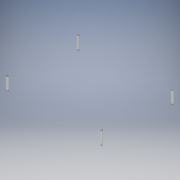
# Autodesk Inventor part: ALU
Saved by Autodesk Inventor 2019 (Build 230136000, 136)
## iProperties
Created: 2020-11-06
Part Number: ALU
Material: Generic
Document SubType Name: Modeling
Designer: james
Density: 1 g/cm^3
Appearance: Default
Author: james
Autodesk Inventor part; units mm, degrees
ref_plane "YZ Plane" through (0, 0, 0) normal (1, 0, 0) x (0, 1, 0)
ref_plane "XZ Plane" through (0, 0, 0) normal (0, 1, 0) x (-1, 0, 0)
ref_plane "XY Plane" through (0, 0, 0) normal (0, 0, 1) x (1, 0, 0)
sketch "Sketch1" plane through (0, 0, 0) normal (0, 1, 0) x (-1, 0, 0)
  line L0 (0, 0) -> (200, 0)
  line L1 (200, 0) -> (200, 152)
  line L2 (200, 152) -> (0, 152)
  line L3 (0, 152) -> (0, 0)
  circle A0 centre (4, 4) radius 0.06
  circle A1 centre (196, 148) radius 0.06
  circle A2 centre (4, 148) radius 0.06
  circle A3 centre (196, 4) radius 0.06
  circle A4 centre (4, 148) radius 1.5
  circle A5 centre (4, 4) radius 1.5
  circle A6 centre (196, 4) radius 1.5
  circle A7 centre (196, 148) radius 1.5
  arc A8 (4, 3.9192) -> (4, 4.0808) centre (4, 4) ccw
  arc A9 (4, 4.0808) -> (4, 3.9192) centre (4, 4) ccw
  arc A10 (196, 147.9192) -> (196, 148.0808) centre (196, 148) ccw
  arc A11 (196, 148.0808) -> (196, 147.9192) centre (196, 148) ccw
  arc A12 (4, 147.9192) -> (4, 148.0808) centre (4, 148) ccw
  arc A13 (4, 148.0808) -> (4, 147.9192) centre (4, 148) ccw
  arc A14 (196, 3.9192) -> (196, 4.0808) centre (196, 4) ccw
  arc A15 (196, 4.0808) -> (196, 3.9192) centre (196, 4) ccw
  arc A16 (4, 147.1992) -> (4, 148.8008) centre (4, 148) ccw
  arc A17 (4, 148.8008) -> (4, 147.1992) centre (4, 148) ccw
  arc A18 (4, 3.1992) -> (4, 4.8008) centre (4, 4) ccw
  arc A19 (4, 4.8008) -> (4, 3.1992) centre (4, 4) ccw
  arc A20 (196, 3.1992) -> (196, 4.8008) centre (196, 4) ccw
  arc A21 (196, 4.8008) -> (196, 3.1992) centre (196, 4) ccw
  arc A22 (196, 147.1992) -> (196, 148.8008) centre (196, 148) ccw
  arc A23 (196, 148.8008) -> (196, 147.1992) centre (196, 148) ccw
  constraints: 32 point on circle, 24 centre point, 8 end point
extrude "Extrusion1" add sketch "Sketch1" along normal blind 25.4 contours A0 | A4 | A5 | A6 | A7 | A9 A8 | A11 A10 | A13 A12 | A15 A14 | A17 A16 | A19 A18 | A21 A20 | A23 A22
body "Solid1"
